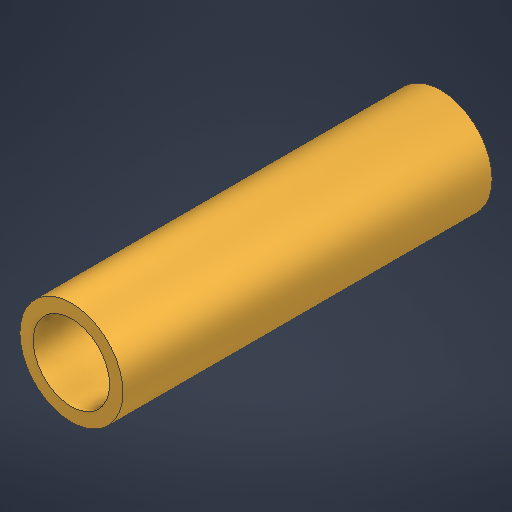
# Autodesk Inventor part: trubicka
Saved by Autodesk Inventor 2025.3 (Build 293356000, 356)
## iProperties
Created: 2025-10-30
Part Number: trubicka
Material: Všeobecné
Document SubType Name: Modeling
Designer: Mr.Happy
Density: 1 g/cm^3
Appearance: Výchozí
Author: Mr.Happy
Autodesk Inventor part; units mm, degrees
ref_plane "YZ Plane" through (0, 0, 0) normal (1, 0, 0) x (0, 1, 0)
ref_plane "XZ Plane" through (0, 0, 0) normal (0, 1, 0) x (-1, 0, 0)
ref_plane "XY Plane" through (0, 0, 0) normal (0, 0, 1) x (1, 0, 0)
sketch "Náčrt1" plane through (0, 0, 0) normal (0, 0, 1) x (1, 0, 0)
  line L0 (0, 7.25) -> (0, -7.25)
  line L1 (1.5, 7.25) -> (2.025, 7.25)
  line L2 (2.025, 7.25) -> (2.025, -7.25)
  line L3 (2.025, -7.25) -> (1.5, -7.25)
  line L4 (1.5, -7.25) -> (1.5, 7.25)
  point P0 (0, 0)
  point P1 (0, 0)
  dimension "d0" = 14.5
  dimension "d1" = 4.05
  dimension "d2" = 3
  constraints: 10 end point, 2 horizontal alignment, 2 parallel, 1 coincident, 1 horizontal, 1 midpoint, 1 perpendicular, 1 vertical
  measures "d0" distance of L0.start L0.end
  measures "d1" diameter of L2 L0
  measures "d2" diameter of L4 L0
revolve "Rotace1" add sketch "Náčrt1" angle 360 about axis through (0, 7.25, 0) along (0, -1, 0)
